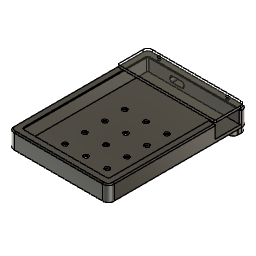
FudaBako (Autodesk Fusion 360 design; units mm, degrees)
Autodesk Fusion 360 part; units mm, degrees
sketch "スケッチ1" plane through (0, 0, 0) normal (0, 0, 1) x (1, 0, 0)
  line L0 (0, 0) -> (72, 0)
  line L1 (72, 0) -> (72, 105.5)
  line L2 (72, 105.5) -> (0, 105.5)
  line L3 (0, 105.5) -> (0, 0)
  line L4 (0, 0) -> (72, 0)
  line L5 (72, 0) -> (72, 85)
  line L6 (72, 85) -> (0, 85)
  line L7 (0, 85) -> (0, 0)
  line L8 (-0.5, -0.5) -> (72.5, -0.5)
  line L9 (72.5, -0.5) -> (72.5, 106)
  line L10 (72.5, 106) -> (-0.5, 106)
  line L11 (-0.5, 106) -> (-0.5, -0.5)
  line L12 (-6.5, -6.5) -> (78.5, -6.5)
  line L13 (78.5, -6.5) -> (78.5, 112)
  line L14 (78.5, 112) -> (-6.5, 112)
  line L15 (-6.5, 112) -> (-6.5, -6.5)
  dimension "d1" = 72
  dimension "d2" = 105.5
  dimension "d3" = 72
  dimension "d4" = 85
  dimension "d5" = 0.5
  dimension "d6" = 0.5
  dimension "d7" = 0.5
  dimension "d8" = 0.5
  dimension "d9" = 6
  dimension "d10" = 6
  dimension "d11" = 6
  dimension "d12" = 6
  constraint horizontal L0
  constraint vertical L1
  constraint horizontal L2
  constraint vertical L3
  constraint coincident L0.start L3.end
  constraint horizontal L4
  constraint vertical L5
  constraint horizontal L6
  constraint vertical L7
  constraint horizontal L8
  constraint vertical L9
  constraint horizontal L10
  constraint vertical L11
  constraint horizontal L12
  constraint vertical L13
  constraint horizontal L14
  constraint vertical L15
  measures "d1" distance of L0.start L0.end
  measures "d2" distance of L0.start L2.end
  measures "d3" distance of L0.start L0.end
  measures "d4" distance of L0.start L6.end
  measures "d5" distance of L2 L10
  measures "d6" distance of L3 L11
  measures "d7" distance of L1 L9
  measures "d8" distance of L4 L8
  measures "d9" distance of L10 L14
  measures "d10" distance of L8 L12
  measures "d11" distance of L9 L13
  measures "d12" distance of L11 L15
extrude "押し出し1" add sketch "スケッチ1" along normal blind 14 contours L12 L13 L14 L15 makes body 1
extrude "押し出し2" add sketch "スケッチ1" 1 faces at (-4.5, 70.5, 0) along normal blind 3 contours L0 L1 L3 L4 L5 L6 L7 | L1 L2 L3 L6 | L8 L9 L10 L11 | L12 L13 L14 L15 on bodies 1 bodies 1
sketch "スケッチ2" plane through (0, 0, 14) normal (0, 0, 1) x (-1, 0, 0)
  line L0 (-72.5, 0.5) -> (0.5, 0.5)
  line L1 (6.5, 6.5) -> (-78.5, 6.5)
  line L2 (-78.5, -112) -> (6.5, -112)
  line L3 (-78.5, -112) -> (6.5, -112)
  line L4 (6.5, -112) -> (6.5, 6.5)
  line L5 (6.5, -85.5) -> (-78.5, -85.5)
  line L6 (-78.5, -85.5) -> (-78.5, -112)
  line L7 (-78.5, -112) -> (6.5, -112)
  line L8 (6.5, -112) -> (6.5, -85.5)
  line L9 (0.5, -106) -> (-72.5, -106)
  line L10 (-72.5, -106) -> (-72.5, -85.5)
  line L11 (-72.5, -85.5) -> (0.5, -85.5)
  line L12 (0.5, -85.5) -> (0.5, -106)
  line L13 (0.5, -106) -> (6.5, -106)
  line L14 (6.5, -106) -> (6.5, -85.5)
  line L15 (6.5, -85.5) -> (0.5, -85.5)
  line L16 (0.5, -85.5) -> (0.5, -106)
  line L17 (-72.5, -106) -> (-78.5, -106)
  line L18 (-78.5, -106) -> (-78.5, -85.5)
  line L19 (-78.5, -85.5) -> (-72.5, -85.5)
  line L20 (-72.5, -85.5) -> (-72.5, -106)
  point P0 (-72.5, -106)
  point P1 (0.5, -106)
  dimension "d190" = 20.5
  constraint coincident L5.start L4
  constraint horizontal L5
  constraint vertical L6
  constraint horizontal L7
  constraint vertical L8
  constraint coincident L2.start L3.start
  constraint horizontal L9
  constraint vertical L10
  constraint horizontal L11
  constraint vertical L12
  constraint coincident L5 L10.end
  constraint coincident P0 L9.end
  constraint coincident P1 L9.start
  constraint horizontal L13
  constraint vertical L14
  constraint horizontal L15
  constraint vertical L16
  constraint horizontal L17
  constraint vertical L18
  constraint horizontal L19
  constraint vertical L20
  measures "d190" distance of P1 L11.end
extrude "押し出し4" cut sketch "スケッチ2" against normal blind 11 contours L5 L6 L10 L17 L18 L19 L20 bodies 1
sketch "スケッチ6" plane through (0, 0, 3) normal (0, 0, 1) x (-1, 0, 0)
  line L0 (0.5, 0.5) -> (-72.5, 0.5)
  line L1 (-72.5, 0.5) -> (-72.5, -85.5)
  line L2 (0.5, -106) -> (0.5, 0.5)
  circle A0 centre (-18, -68) radius 1.1
  line L3 (-72, -85) -> (0, -85)
  line L4 (0, -105.5) -> (0, 0)
  circle A1 centre (-54, -68) radius 1.1
  line L5 (-72, 0) -> (-72, -85)
  circle A2 centre (-36, -51) radius 1.1
  circle A3 centre (-18, -51) radius 1.1
  circle A4 centre (-54, -51) radius 1.1
  circle A5 centre (-36, -68) radius 1.1
  circle A6 centre (-18, -34) radius 1.1
  circle A7 centre (-36, -34) radius 1.1
  circle A8 centre (-54, -34) radius 1.1
  circle A9 centre (-36, -17) radius 1.1
  circle A10 centre (-18, -17) radius 1.1
  circle A11 centre (-54, -17) radius 1.1
  line L6 (0, -85) -> (0, 0)
  line L7 (0, 0) -> (-72, 0)
  circle A12 centre (-56.5, -4) radius 1.1
  line L8 (-72.5, -85.5) -> (-78.5, -85.5)
  line L9 (-78.5, -85.5) -> (-78.5, -106)
  line L10 (-78.5, -106) -> (0.5, -106)
  circle A13 centre (-15.5, -4) radius 1.1
  dimension "d45" = 2.2
  dimension "d46" = 17
  dimension "d47" = 18
  dimension "d48" = 2.2
  dimension "d49" = 17
  dimension "d50" = 18
  dimension "d51" = 2.2
  dimension "d52" = 34
  dimension "d53" = 36
  dimension "d54" = 2.2
  dimension "d55" = 18
  dimension "d56" = 34
  dimension "d57" = 2.2
  dimension "d58" = 2.2
  dimension "d59" = 17
  dimension "d60" = 36
  dimension "d61" = 18
  dimension "d62" = 34
  dimension "d63" = 2.2
  dimension "d64" = 2.2
  dimension "d65" = 2.2
  dimension "d66" = 2.2
  dimension "d67" = 2.2
  dimension "d68" = 2.2
  dimension "d69" = 18
  dimension "d70" = 36
  dimension "d71" = 18
  dimension "d72" = 34
  dimension "d73" = 17
  dimension "d74" = 18
  dimension "d75" = 36
  dimension "d76" = 17
  dimension "d77" = 34
  dimension "d78" = 34
  dimension "d79" = 18
  dimension "d80" = 17
  dimension "d81" = 2.2
  dimension "d82" = 15.5
  dimension "d83" = 4
  dimension "d268" = 2.2
  dimension "d269" = 15.5
  dimension "d270" = 4
  measures "d45" diameter of A0
  measures "d46" distance of A0.centre L3
  measures "d47" distance of A0.centre L4
  measures "d48" diameter of A1
  measures "d49" distance of L3 A1.centre
  measures "d50" distance of A1.centre L5
  measures "d51" diameter of A2
  measures "d52" distance of L3 A2.centre
  measures "d53" distance of L4 A2.centre
  measures "d54" diameter of A3
  measures "d55" distance of L4 A3.centre
  measures "d56" distance of L3 A3.centre
  measures "d57" diameter of A4
  measures "d58" diameter of A5
  measures "d59" distance of L3 A5.centre
  measures "d60" distance of L4 A5.centre
  measures "d61" distance of L5 A4.centre
  measures "d62" distance of L3 A4.centre
  measures "d63" diameter of A7
  measures "d64" diameter of A6
  measures "d65" diameter of A8
  measures "d66" diameter of A9
  measures "d67" diameter of A10
  measures "d68" diameter of A11
  measures "d69" distance of L5 A8.centre
  measures "d70" distance of A7.centre L6
  measures "d71" distance of A6.centre L6
  measures "d72" distance of A6.centre L7
  measures "d73" distance of A10.centre L7
  measures "d74" distance of A10.centre L6
  measures "d75" distance of A9.centre L6
  measures "d76" distance of A9.centre L7
  measures "d77" distance of A7.centre L7
  measures "d78" distance of A8.centre L7
  measures "d79" distance of L5 A11.centre
  measures "d80" distance of A11.centre L7
  measures "d81" diameter of A12
  measures "d82" distance of L5 A12.centre
  measures "d83" distance of L7 A12.centre
  measures "d268" diameter of A13
  measures "d269" distance of L6 A13.centre
  measures "d270" distance of L7 A13.centre
extrude "押し出し8" cut sketch "スケッチ6" against normal blind 3 contours A0 | A1 | A2 | A3 | A4 | A5 | A6 | A7 | A8 | A9 | A10 | A11 | A12 | A13 bodies 1
sketch "スケッチ7" plane through (0, 0, 3) normal (0, 0, 1) x (-1, 0, 0)
  circle A0 centre (-54, -17) radius 1.1
  circle A1 centre (-18, -34) radius 1.1
  circle A2 centre (-54, -68) radius 1.1
  circle A3 centre (-36, -68) radius 1.1
  circle A4 centre (-18, -51) radius 1.1
  circle A5 centre (-36, -17) radius 1.1
  circle A6 centre (-54, -34) radius 1.1
  circle A7 centre (-36, -34) radius 1.1
  circle A8 centre (-54, -51) radius 1.1
  circle A9 centre (-18, -68) radius 1.1
  circle A10 centre (-36, -51) radius 1.1
  circle A11 centre (-18, -17) radius 1.1
  circle A12 centre (-56.5, -4) radius 1.1
  line L0 (0.5, 0.5) -> (-72.5, 0.5)
  line L1 (-72.5, 0.5) -> (-72.5, -85.5)
  line L2 (0.5, -106) -> (0.5, 0.5)
  circle A13 centre (-18, -68) radius 2.1
  circle A14 centre (-36, -68) radius 2.1
  circle A15 centre (-54, -68) radius 2.1
  circle A16 centre (-18, -51) radius 2.1
  circle A17 centre (-36, -51) radius 2.1
  circle A18 centre (-54, -51) radius 2.1
  circle A19 centre (-54, -34) radius 2.1
  circle A20 centre (-54, -17) radius 2.1
  circle A21 centre (-56.5, -4) radius 2.1
  circle A22 centre (-36, -34) radius 2.1
  circle A23 centre (-18, -34) radius 2.1
  circle A24 centre (-18, -17) radius 2.1
  circle A25 centre (-36, -17) radius 2.1
  line L3 (-72.5, -85.5) -> (-78.5, -85.5)
  line L4 (-78.5, -85.5) -> (-78.5, -106)
  line L5 (-78.5, -106) -> (0.5, -106)
  circle A26 centre (-15.5, -4) radius 1.1
  circle A27 centre (-15.5, -4) radius 2.1
  dimension "d86" = 4.2
  dimension "d87" = 4.2
  dimension "d88" = 4.2
  dimension "d89" = 4.2
  dimension "d90" = 4.2
  dimension "d91" = 4.2
  dimension "d92" = 4.2
  dimension "d93" = 4.2
  dimension "d94" = 4.2
  dimension "d95" = 4.2
  dimension "d96" = 4.2
  dimension "d97" = 4.2
  dimension "d98" = 4.2
  dimension "d272" = 4.2
  constraint concentric A9 A13
  constraint concentric A3 A14
  constraint concentric A2 A15
  constraint concentric A4 A16
  constraint concentric A10 A17
  constraint concentric A8 A18
  constraint concentric A6 A19
  constraint concentric A0 A20
  constraint concentric A12 A21
  constraint concentric A7 A22
  constraint concentric A1 A23
  constraint concentric A11 A24
  constraint concentric A5 A25
  constraint concentric A26 A27
  measures "d86" diameter of A13
  measures "d87" diameter of A14
  measures "d88" diameter of A15
  measures "d89" diameter of A16
  measures "d90" diameter of A17
  measures "d91" diameter of A18
  measures "d92" diameter of A19
  measures "d93" diameter of A20
  measures "d94" diameter of A21
  measures "d95" diameter of A22
  measures "d96" diameter of A23
  measures "d97" diameter of A24
  measures "d98" diameter of A25
  measures "d272" diameter of A27
extrude "押し出し9" cut sketch "スケッチ7" against normal blind 1 contours A13 | A14 | A15 | A16 | A17 | A18 | A19 | A20 | A21 | A22 | A23 | A24 | A25 | A27 bodies 1
sketch "スケッチ8" plane through (0, 0, 0) normal (0, 0, 1) x (1, 0, 0)
  circle A0 centre (72.5, -0.5) radius 3.75
  line L0 (78.5, -6.5) -> (78.5, 112)
  line L1 (-6.5, -6.5) -> (78.5, -6.5)
  circle A1 centre (-0.5, -0.5) radius 3.75
  line L2 (-6.5, 112) -> (-6.5, -6.5)
  circle A2 centre (72.5, 106) radius 3.75
  line L3 (78.5, 112) -> (-6.5, 112)
  circle A3 centre (-0.5, 106) radius 3.75
  dimension "d101" = 7.5
  dimension "d102" = 6
  dimension "d103" = 6
  dimension "d104" = 7.5
  dimension "d105" = 6
  dimension "d106" = 6
  dimension "d107" = 7.5
  dimension "d108" = 6
  dimension "d109" = 6
  dimension "d110" = 7.5
  dimension "d111" = 6
  dimension "d112" = 6
  measures "d101" diameter of A0
  measures "d102" distance of A0.centre L0
  measures "d103" distance of A0.centre L1
  measures "d104" diameter of A1
  measures "d105" distance of L1 A1.centre
  measures "d106" distance of A1.centre L2
  measures "d107" diameter of A2
  measures "d108" distance of L0 A2.centre
  measures "d109" distance of A2.centre L3
  measures "d110" diameter of A3
  measures "d111" distance of L2 A3.centre
  measures "d112" distance of L3 A3.centre
extrude "押し出し10" cut sketch "スケッチ8" along normal blind 0.5 contours A0 | A1 | A2 | A3 bodies 1
sketch "スケッチ10" plane through (0, 0, 0) normal (0, 0, -1) x (1, 0, 0)
  circle A0 centre (56.5, -4) radius 1.1
  circle A1 centre (18, -17) radius 1.1
  circle A2 centre (36, -51) radius 1.1
  circle A3 centre (18, -68) radius 1.1
  circle A4 centre (54, -51) radius 1.1
  circle A5 centre (36, -34) radius 1.1
  circle A6 centre (54, -34) radius 1.1
  circle A7 centre (36, -17) radius 1.1
  circle A8 centre (18, -51) radius 1.1
  circle A9 centre (36, -68) radius 1.1
  circle A10 centre (54, -68) radius 1.1
  circle A11 centre (18, -34) radius 1.1
  circle A12 centre (54, -17) radius 1.1
  circle A13 centre (72.5, 0.5) radius 3.75
  circle A14 centre (-0.5, 0.5) radius 3.75
  circle A15 centre (56.5, -4) radius 2
  circle A16 centre (54, -17) radius 2
  circle A17 centre (36, -17) radius 2
  circle A18 centre (18, -17) radius 2
  circle A19 centre (18, -34) radius 2
  circle A20 centre (36, -34) radius 2
  circle A21 centre (54, -34) radius 2
  circle A22 centre (54, -51) radius 2
  circle A23 centre (36, -51) radius 2
  circle A24 centre (18, -51) radius 2
  circle A25 centre (18, -68) radius 2
  circle A26 centre (36, -68) radius 2
  circle A27 centre (54, -68) radius 2
  line L0 (-6.5, 6.5) -> (-6.5, -112)
  line L1 (78.5, -112) -> (78.5, 6.5)
  line L2 (78.5, 6.5) -> (-6.5, 6.5)
  circle A28 centre (-0.5, -106) radius 3.75
  circle A29 centre (72.5, -106) radius 3.75
  line L3 (-6.5, -112) -> (78.5, -112)
  circle A30 centre (15.5, -4) radius 1.1
  circle A31 centre (15.5, -4) radius 2
  dimension "d135" = 4
  dimension "d136" = 4
  dimension "d137" = 4
  dimension "d138" = 4
  dimension "d139" = 4
  dimension "d140" = 4
  dimension "d141" = 4
  dimension "d142" = 4
  dimension "d143" = 4
  dimension "d144" = 4
  dimension "d145" = 4
  dimension "d146" = 4
  dimension "d147" = 4
  dimension "d271" = 4
  constraint concentric A0 A15
  constraint concentric A12 A16
  constraint concentric A7 A17
  constraint concentric A1 A18
  constraint concentric A11 A19
  constraint concentric A5 A20
  constraint concentric A6 A21
  constraint concentric A4 A22
  constraint concentric A2 A23
  constraint concentric A8 A24
  constraint concentric A3 A25
  constraint concentric A9 A26
  constraint concentric A10 A27
  constraint concentric A30 A31
  measures "d135" diameter of A15
  measures "d136" diameter of A16
  measures "d137" diameter of A17
  measures "d138" diameter of A18
  measures "d139" diameter of A19
  measures "d140" diameter of A20
  measures "d141" diameter of A21
  measures "d142" diameter of A22
  measures "d143" diameter of A23
  measures "d144" diameter of A24
  measures "d145" diameter of A25
  measures "d146" diameter of A26
  measures "d147" diameter of A27
  measures "d271" diameter of A31
extrude "押し出し13" cut sketch "スケッチ10" against normal blind 0.5 contours A15 | A16 | A17 | A18 | A19 | A20 | A21 | A22 | A23 | A24 | A25 | A26 | A27 | A31 bodies 1
fillet "フィレット4" radius 1 2 edges at (72.5, -0.5, 8.5) (-0.5, -0.5, 8.5) on bodies 1
fillet "フィレット16" radius 1 1 edges at (-0.5, 106, 8.5) on bodies 1
chamfer "面取り12" distance 0.5 angle 45 5 edges at (72.5, 43, 14) (72.2071, -0.2071, 14) (36, -0.5, 14) (-0.2071, -0.2071, 14) (-0.5, 53.25, 14) on bodies 1
fillet "フィレット5" radius 5 curvature continuous 2 edges at (78.5, -6.5, 7) (-6.5, -6.5, 7) on bodies 1
fillet "フィレット8" radius 1 1 edges at (78.5, 85.5, 8.5) on bodies 1
fillet "フィレット13" radius 5 curvature continuous 2 edges at (78.5, 112, 7) (-6.5, 112, 7) on bodies 1
chamfer "面取り21" distance 1 angle 45 12 edges at (36, 112, 14) (77.0839, 110.8219, 14) (78.5, 106.75, 14) (78.5, 41.5, 14) (75.25, 85.5, 14) (78.2071, 85.2071, 14) (78.5, 41.5, 14) (77.3219, -5.0839, 14) (36, -6.5, 14) (-5.0839, -5.3219, 14) (-6.5, 52.75, 14) (-5.3219, 110.5839, 14) on bodies 1
fillet "フィレット15" radius 1 2 edges at (72.5, 85.5, 8) (78.5, 106, 8) on bodies 1
sketch "スケッチ17" plane through (0, 0, 14) normal (0, 0, 1) x (-1, 0, 0)
  line L0 (-77.5, -106.5) -> (-77.5, -107)
  line L1 (-73.5, -111) -> (1.5, -111)
  line L2 (5.5, -107) -> (5.5, 1.5)
  circle A0 centre (-7, -108.5) radius 0.9
  circle A1 centre (-65, -108.5) radius 0.9
  line L3 (-73.5, -112) -> (1.5, -112)
  spline S0 degree 3 poles (-73.5, -111) (-73.8454, -111) (-74.1654, -110.9986) (-74.7027, -110.9408) (-74.9267, -110.8989) (-75.2988, -110.7824) (-75.4373, -110.7274) (-75.8631, -110.522) (-76.1365, -110.3374) (-76.4029, -110.0896) (-76.6724, -109.839) (-76.9308, -109.521) (-77.3045, -108.8015) (-77.3918, -108.4745) (-77.4569, -108.0594) (-77.4694, -107.9483) (-77.4991, -107.5718) (-77.5, -107.2964) (-77.5, -107) knots 0 0 0 0 0.103632 0.103632 0.182254 0.182254 0.2323 0.2323 0.339984 0.339984 0.339984 0.448922 0.448922 0.55397 0.55397 0.591904 0.591904 0.679968 0.679968 0.679968 0.679968
  spline S1 degree 3 poles (5.5, -107) (5.5, -107.3454) (5.4986, -107.6654) (5.4408, -108.2027) (5.3989, -108.4267) (5.2824, -108.7988) (5.2274, -108.9373) (5.022, -109.3631) (4.8374, -109.6365) (4.5896, -109.9029) (4.339, -110.1724) (4.021, -110.4308) (3.3015, -110.8045) (2.9745, -110.8918) (2.5594, -110.9569) (2.4483, -110.9694) (2.0718, -110.9991) (1.7964, -111) (1.5, -111) knots 0 0 0 0 0.103632 0.103632 0.182254 0.182254 0.2323 0.2323 0.339984 0.339984 0.339984 0.448922 0.448922 0.55397 0.55397 0.591904 0.591904 0.679968 0.679968 0.679968 0.679968
  line L4 (1, -0.5) -> (1, -105)
  spline S2 degree 3 poles (1.5, 5.5) (1.8454, 5.5) (2.1654, 5.4986) (2.7027, 5.4408) (2.9267, 5.3989) (3.2988, 5.2824) (3.4373, 5.2274) (3.8631, 5.022) (4.1365, 4.8374) (4.4029, 4.5896) (4.6724, 4.339) (4.9308, 4.021) (5.3045, 3.3015) (5.3918, 2.9745) (5.4569, 2.5594) (5.4694, 2.4483) (5.4991, 2.0718) (5.5, 1.7964) (5.5, 1.5) knots 0 0 0 0 0.103632 0.103632 0.182254 0.182254 0.2323 0.2323 0.339984 0.339984 0.339984 0.448922 0.448922 0.55397 0.55397 0.591904 0.591904 0.679968 0.679968 0.679968 0.679968
  line L5 (1.5, 5.5) -> (-73.5, 5.5)
  spline S3 degree 3 poles (-77.5, 1.5) (-77.5, 1.8454) (-77.4986, 2.1654) (-77.4408, 2.7027) (-77.3989, 2.9267) (-77.2824, 3.2988) (-77.2274, 3.4373) (-77.022, 3.8631) (-76.8374, 4.1365) (-76.5896, 4.4029) (-76.339, 4.6724) (-76.021, 4.9308) (-75.3015, 5.3045) (-74.9745, 5.3918) (-74.5594, 5.4569) (-74.4483, 5.4694) (-74.0718, 5.4991) (-73.7964, 5.5) (-73.5, 5.5) knots 0 0 0 0 0.103632 0.103632 0.182254 0.182254 0.2323 0.2323 0.339984 0.339984 0.339984 0.448922 0.448922 0.55397 0.55397 0.591904 0.591904 0.679968 0.679968 0.679968 0.679968
  line L6 (-77.5, 1.5) -> (-77.5, -84.5)
  line L7 (-77.5, -84.5) -> (-73, -84.5)
  line L8 (-73, -84.5) -> (-73, -0.5)
  arc A2 (-71.5, 1) -> (-73, -0.5) centre (-71.5, -0.5) ccw
  line L9 (-71.5, 1) -> (-0.5, 1)
  arc A3 (1, -0.5) -> (-0.5, 1) centre (-0.5, -0.5) ccw
  arc A4 (-0.5, -106.5) -> (1, -105) centre (-0.5, -105) ccw
  line L10 (-0.5, -106.5) -> (-77.5, -106.5)
  point P0 (-78.5, -107)
  point P1 (6.5, -107)
  dimension "d236" = 1.8
  dimension "d237" = 1.8
  dimension "d238" = 13.5
  dimension "d240" = 3.5
  dimension "d241" = 3.5
  measures "d236" diameter of A0
  measures "d237" diameter of A1
  measures "d238" horizontal distance of A1.centre P0
  measures "d240" distance of A0.centre L3
  measures "d241" distance of A1.centre L3
extrude "押し出し22" cut sketch "スケッチ17" against normal blind 6 contours A0 | A1 bodies 1
sketch "スケッチ18" plane through (0, 112, 0) normal (0, 1, 0) x (-1, 0, 0)
  line L0 (1.5, 13) -> (-73.5, 13)
  line L1 (-73.5, 13) -> (-73.5, 0)
  line L2 (-73.5, 0) -> (1.5, 0)
  line L3 (1.5, 0) -> (1.5, 13)
  line L4 (-51.5, 10.1) -> (-43.5, 10.1)
  line L5 (-41.5, 8.1) -> (-41.5, 7.1)
  line L6 (-43.5, 5.1) -> (-51.5, 5.1)
  line L7 (-53.5, 7.1) -> (-53.5, 8.1)
  line L8 (-28.5, 10.1) -> (-20.5, 10.1)
  line L9 (-18.5, 8.1) -> (-18.5, 7.1)
  line L10 (-20.5, 5.1) -> (-28.5, 5.1)
  line L11 (-30.5, 7.1) -> (-30.5, 8.1)
  line L12 (-78.5, 13) -> (-78.5, 3)
  arc A0 (-51.5, 10.1) -> (-53.5, 8.1) centre (-51.5, 8.1) ccw
  arc A1 (-53.5, 7.1) -> (-51.5, 5.1) centre (-51.5, 7.1) ccw
  arc A2 (-41.5, 8.1) -> (-43.5, 10.1) centre (-43.5, 8.1) ccw
  arc A3 (-43.5, 5.1) -> (-41.5, 7.1) centre (-43.5, 7.1) ccw
  arc A4 (-28.5, 10.1) -> (-30.5, 8.1) centre (-28.5, 8.1) ccw
  arc A5 (-30.5, 7.1) -> (-28.5, 5.1) centre (-28.5, 7.1) ccw
  arc A6 (-18.5, 8.1) -> (-20.5, 10.1) centre (-20.5, 8.1) ccw
  arc A7 (-20.5, 5.1) -> (-18.5, 7.1) centre (-20.5, 7.1) ccw
  line L13 (6.5, 0) -> (6.5, 13)
  point P0 (-53.5, 10.1)
  point P1 (-41.5, 10.1)
  point P2 (-53.5, 5.1)
  point P3 (-30.5, 10.1)
  point P4 (-18.5, 10.1)
  point P5 (-18.5, 5.1)
  point P6 (-30.5, 5.1)
  dimension "d244" = 25
  dimension "d246" = 12
  dimension "d247" = 12
  dimension "d248" = 5
  dimension "d249" = 5
  dimension "d250" = 5.1
  dimension "d251" = 5.1
  dimension "d252" = 2
  dimension "d253" = 2
  dimension "d254" = 2
  dimension "d255" = 2
  dimension "d256" = 2
  dimension "d257" = 2
  dimension "d258" = 2
  dimension "d259" = 2
  dimension "d282" = 25
  constraint horizontal L4
  constraint vertical L5
  constraint horizontal L6
  constraint vertical L7
  constraint horizontal L8
  constraint vertical L9
  constraint horizontal L10
  constraint vertical L11
  constraint coincident P0 L4
  constraint coincident P0 L7
  constraint tangent L4 A0
  constraint tangent L7 A0
  constraint coincident P2 L6
  constraint coincident P2 L7
  constraint tangent L6 A1
  constraint tangent L7 A1
  constraint coincident P1 L4
  constraint coincident P1 L5
  constraint tangent L4 A2
  constraint tangent L5 A2
  constraint tangent L5 A3
  constraint tangent L6 A3
  constraint coincident P3 L8
  constraint coincident P3 L11
  constraint tangent L8 A4
  constraint tangent L11 A4
  constraint coincident P6 L10
  constraint coincident P6 L11
  constraint tangent L10 A5
  constraint tangent L11 A5
  constraint coincident P4 L8
  constraint coincident P4 L9
  constraint tangent L8 A6
  constraint tangent L9 A6
  constraint coincident P5 L9
  constraint coincident P5 L10
  constraint tangent L9 A7
  constraint tangent L10 A7
  measures "d244" distance of L7 L12
  measures "d246" distance of P3 P4
  measures "d247" distance of P0 P1
  measures "d248" distance of P0 P2
  measures "d249" distance of P4 P5
  measures "d250" distance of L2 P6
  measures "d251" distance of L2 P2
  measures "d252" radius of A0
  measures "d253" radius of A1
  measures "d254" radius of A2
  measures "d255" radius of A3
  measures "d256" radius of A4
  measures "d257" radius of A5
  measures "d258" radius of A6
  measures "d259" radius of A7
  measures "d282" distance of L9.start L13
extrude "押し出し23" cut sketch "スケッチ18" against normal blind 7 contours L8 L9 L10 L11 A4 A5 A6 A7 bodies 1
chamfer "面取り22" distance 1 angle 45 8 edges at (24.5, 112, 10.1) (19.0858, 112, 9.5142) (18.5, 112, 7.6) (19.0858, 112, 5.6858) (24.5, 112, 5.1) (29.9142, 112, 5.6858) (30.5, 112, 7.6) (29.9142, 112, 9.5142) on bodies 1
sketch "スケッチ19" plane through (0, 0, 14) normal (0, 0, 1) x (-1, 0, 0)
  circle A0 centre (-7, -108.5) radius 0.9
  circle A1 centre (-65, -108.5) radius 0.9
  line L0 (-77.5, -106.5) -> (-77.5, -107)
  line L1 (-73.5, -111) -> (1.5, -111)
  line L2 (5.5, -107) -> (5.5, 1.5)
  line L3 (5.5, -107) -> (-77.5, -107)
  line L4 (-77.5, -107) -> (-77.5, -86.5)
  line L5 (-76.5, -85.5) -> (4.5, -85.5)
  line L6 (5.5, -86.5) -> (5.5, -107)
  arc A2 (-76.5, -85.5) -> (-77.5, -86.5) centre (-76.5, -86.5) ccw
  arc A3 (5.5, -86.5) -> (4.5, -85.5) centre (4.5, -86.5) ccw
  spline S0 degree 3 poles (-73.5, -111) (-73.8454, -111) (-74.1654, -110.9986) (-74.7027, -110.9408) (-74.9267, -110.8989) (-75.2988, -110.7824) (-75.4373, -110.7274) (-75.8631, -110.522) (-76.1365, -110.3374) (-76.4029, -110.0896) (-76.6724, -109.839) (-76.9308, -109.521) (-77.3045, -108.8015) (-77.3918, -108.4745) (-77.4569, -108.0594) (-77.4694, -107.9483) (-77.4991, -107.5718) (-77.5, -107.2964) (-77.5, -107) knots 0 0 0 0 0.103632 0.103632 0.182254 0.182254 0.2323 0.2323 0.339984 0.339984 0.339984 0.448922 0.448922 0.55397 0.55397 0.591904 0.591904 0.679968 0.679968 0.679968 0.679968
  spline S1 degree 3 poles (5.5, -107) (5.5, -107.3454) (5.4986, -107.6654) (5.4408, -108.2027) (5.3989, -108.4267) (5.2824, -108.7988) (5.2274, -108.9373) (5.022, -109.3631) (4.8374, -109.6365) (4.5896, -109.9029) (4.339, -110.1724) (4.021, -110.4308) (3.3015, -110.8045) (2.9745, -110.8918) (2.5594, -110.9569) (2.4483, -110.9694) (2.0718, -110.9991) (1.7964, -111) (1.5, -111) knots 0 0 0 0 0.103632 0.103632 0.182254 0.182254 0.2323 0.2323 0.339984 0.339984 0.339984 0.448922 0.448922 0.55397 0.55397 0.591904 0.591904 0.679968 0.679968 0.679968 0.679968
  line L7 (1, -0.5) -> (1, -105)
  spline S2 degree 3 poles (1.5, 5.5) (1.8454, 5.5) (2.1654, 5.4986) (2.7027, 5.4408) (2.9267, 5.3989) (3.2988, 5.2824) (3.4373, 5.2274) (3.8631, 5.022) (4.1365, 4.8374) (4.4029, 4.5896) (4.6724, 4.339) (4.9308, 4.021) (5.3045, 3.3015) (5.3918, 2.9745) (5.4569, 2.5594) (5.4694, 2.4483) (5.4991, 2.0718) (5.5, 1.7964) (5.5, 1.5) knots 0 0 0 0 0.103632 0.103632 0.182254 0.182254 0.2323 0.2323 0.339984 0.339984 0.339984 0.448922 0.448922 0.55397 0.55397 0.591904 0.591904 0.679968 0.679968 0.679968 0.679968
  line L8 (1.5, 5.5) -> (-73.5, 5.5)
  spline S3 degree 3 poles (-77.5, 1.5) (-77.5, 1.8454) (-77.4986, 2.1654) (-77.4408, 2.7027) (-77.3989, 2.9267) (-77.2824, 3.2988) (-77.2274, 3.4373) (-77.022, 3.8631) (-76.8374, 4.1365) (-76.5896, 4.4029) (-76.339, 4.6724) (-76.021, 4.9308) (-75.3015, 5.3045) (-74.9745, 5.3918) (-74.5594, 5.4569) (-74.4483, 5.4694) (-74.0718, 5.4991) (-73.7964, 5.5) (-73.5, 5.5) knots 0 0 0 0 0.103632 0.103632 0.182254 0.182254 0.2323 0.2323 0.339984 0.339984 0.339984 0.448922 0.448922 0.55397 0.55397 0.591904 0.591904 0.679968 0.679968 0.679968 0.679968
  line L9 (-77.5, 1.5) -> (-77.5, -84.5)
  line L10 (-77.5, -84.5) -> (-73, -84.5)
  line L11 (-73, -84.5) -> (-73, -0.5)
  arc A4 (-71.5, 1) -> (-73, -0.5) centre (-71.5, -0.5) ccw
  line L12 (-71.5, 1) -> (-0.5, 1)
  arc A5 (1, -0.5) -> (-0.5, 1) centre (-0.5, -0.5) ccw
  arc A6 (-0.5, -106.5) -> (1, -105) centre (-0.5, -105) ccw
  line L13 (-0.5, -106.5) -> (-77.5, -106.5)
  dimension "d264" = 1
  dimension "d265" = 1
  constraint horizontal L3
  constraint vertical L4
  constraint horizontal L5
  constraint vertical L6
  constraint coincident L0.start L4
  constraint coincident L2.start L3
  constraint tangent L4 A2
  constraint tangent L5 A2
  constraint tangent L5 A3
  constraint tangent L6 A3
  measures "d264" radius of A2
  measures "d265" radius of A3
extrude "押し出し24" add sketch "スケッチ19" along normal blind 2 separate body contours L0 L2 L3 L4 L5 L6 A3 L7 A6 L13 | L4 L5 A2 L7 A6 L13 | L1 L3 S0 S1 makes body 2
sketch "スケッチ20" plane through (0, 0, 0) normal (0, 0, -1) x (1, 0, 0)
  line L0 (-1.5, -112) -> (73.5, -112)
  line L1 (78.5, -107) -> (78.5, 1.5)
  line L2 (73.5, 6.5) -> (-1.5, 6.5)
  line L3 (-6.5, 1.5) -> (-6.5, -107)
  circle A0 centre (72.5, 0.5) radius 3.75
  circle A1 centre (72.5, -106) radius 3.75
  circle A2 centre (-0.5, 0.5) radius 3.75
  circle A3 centre (-0.5, -106) radius 3.75
  circle A4 centre (15.5, -4) radius 2
  circle A5 centre (18, -51) radius 2
  circle A6 centre (36, -34) radius 2
  circle A7 centre (54, -17) radius 2
  circle A8 centre (36, -17) radius 2
  circle A9 centre (54, -34) radius 2
  circle A10 centre (18, -68) radius 2
  circle A11 centre (54, -68) radius 2
  circle A12 centre (36, -51) radius 2
  circle A13 centre (18, -34) radius 2
  circle A14 centre (56.5, -4) radius 2
  circle A15 centre (18, -17) radius 2
  circle A16 centre (54, -51) radius 2
  circle A17 centre (36, -68) radius 2
  circle A18 centre (58.5, -108.5) radius 0.9
  circle A19 centre (13.5, -108.5) radius 0.9
  spline S0 degree 3 poles (73.5, 6.5) (74.1075, 6.5) (74.7567, 6.5) (75.9834, 6.1158) (76.4633, 5.8499) (77.3109, 5.1398) (77.7145, 4.6816) (78.2502, 3.6503) (78.3672, 3.2095) (78.5, 2.3629) (78.5, 1.9241) (78.5, 1.5) knots 0 0 0 0 0.182254 0.182254 0.32114 0.32114 0.448922 0.448922 0.55397 0.55397 0.679968 0.679968 0.679968 0.679968
  spline S1 degree 3 poles (-6.5, 1.5) (-6.5, 2.1075) (-6.5, 2.7567) (-6.1158, 3.9834) (-5.8499, 4.4633) (-5.1398, 5.3109) (-4.6816, 5.7145) (-3.6503, 6.2502) (-3.2095, 6.3672) (-2.3629, 6.5) (-1.9241, 6.5) (-1.5, 6.5) knots 0 0 0 0 0.182254 0.182254 0.32114 0.32114 0.448922 0.448922 0.55397 0.55397 0.679968 0.679968 0.679968 0.679968
  spline S2 degree 3 poles (-1.5, -112) (-2.1075, -112) (-2.7567, -112) (-3.9834, -111.6158) (-4.4633, -111.3499) (-5.3109, -110.6398) (-5.7145, -110.1816) (-6.2502, -109.1503) (-6.3672, -108.7095) (-6.5, -107.8629) (-6.5, -107.4241) (-6.5, -107) knots 0 0 0 0 0.182254 0.182254 0.32114 0.32114 0.448922 0.448922 0.55397 0.55397 0.679968 0.679968 0.679968 0.679968
  spline S3 degree 3 poles (78.5, -107) (78.5, -107.6075) (78.5, -108.2567) (78.1158, -109.4834) (77.8499, -109.9633) (77.1398, -110.8109) (76.6816, -111.2145) (75.6503, -111.7502) (75.2095, -111.8672) (74.3629, -112) (73.9241, -112) (73.5, -112) knots 0 0 0 0 0.182254 0.182254 0.32114 0.32114 0.448922 0.448922 0.55397 0.55397 0.679968 0.679968 0.679968 0.679968
  dimension "d273" = 1.8
  dimension "d274" = 1.8
  dimension "d277" = 3.5
  dimension "d278" = 3.5
  dimension "d289" = 20
  dimension "d290" = 20
  measures "d273" diameter of A18
  measures "d274" diameter of A19
  measures "d277" distance of L0 A18.centre
  measures "d278" distance of L0 A19.centre
  measures "d289" horizontal distance of L3.end A19.centre
  measures "d290" horizontal distance of L1.start A18.centre
extrude "押し出し25" cut sketch "スケッチ20" against normal blind 6 contours A18 | A19 bodies 1
chamfer "面取り23" distance 0.5 angle 45 8 edges at (36, 112, 0) (-5.0839, 110.8219, 0) (-6.5, 52.75, 0) (-5.3219, -5.0839, 0) (36, -6.5, 0) (77.0839, -5.3219, 0) (78.5, 52.75, 0) (77.3219, 110.5839, 0) on bodies 1
sketch "スケッチ21" plane through (0, 0, 16) normal (0, 0, 1) x (-1, 0, 0)
  circle A0 centre (-7, -108.5) radius 0.9
  circle A1 centre (-65, -108.5) radius 0.9
  arc A2 (5.5, -86.5) -> (4.5, -85.5) centre (4.5, -86.5) ccw
  line L0 (4.5, -85.5) -> (-76.5, -85.5)
  arc A3 (-76.5, -85.5) -> (-77.5, -86.5) centre (-76.5, -86.5) ccw
  line L1 (-77.5, -86.5) -> (-77.5, -107)
  spline S0 degree 3 poles (-77.5, -107) (-77.5, -107.2964) (-77.4991, -107.5718) (-77.4694, -107.9483) (-77.4569, -108.0594) (-77.3918, -108.4745) (-77.3045, -108.8015) (-76.9308, -109.521) (-76.6724, -109.839) (-76.4029, -110.0896) (-76.1365, -110.3374) (-75.8631, -110.522) (-75.4373, -110.7274) (-75.2988, -110.7824) (-74.9267, -110.8989) (-74.7027, -110.9408) (-74.1654, -110.9986) (-73.8454, -111) (-73.5, -111) knots -0.679968 -0.679968 -0.679968 -0.679968 -0.591904 -0.591904 -0.55397 -0.55397 -0.448922 -0.448922 -0.339984 -0.339984 -0.339984 -0.2323 -0.2323 -0.182254 -0.182254 -0.103632 -0.103632 0 0 0 0
  line L2 (-73.5, -111) -> (1.5, -111)
  spline S1 degree 3 poles (1.5, -111) (1.7964, -111) (2.0718, -110.9991) (2.4483, -110.9694) (2.5594, -110.9569) (2.9745, -110.8918) (3.3015, -110.8045) (4.021, -110.4308) (4.339, -110.1724) (4.5896, -109.9029) (4.8374, -109.6365) (5.022, -109.3631) (5.2274, -108.9373) (5.2824, -108.7988) (5.3989, -108.4267) (5.4408, -108.2027) (5.4986, -107.6654) (5.5, -107.3454) (5.5, -107) knots -0.679968 -0.679968 -0.679968 -0.679968 -0.591904 -0.591904 -0.55397 -0.55397 -0.448922 -0.448922 -0.339984 -0.339984 -0.339984 -0.2323 -0.2323 -0.182254 -0.182254 -0.103632 -0.103632 0 0 0 0
  line L3 (5.5, -107) -> (5.5, -86.5)
  circle A4 centre (-7, -108.5) radius 1.1
  circle A5 centre (-65, -108.5) radius 1.1
  dimension "d285" = 2.2
  dimension "d286" = 2.2
  constraint concentric A0 A4
  constraint concentric A1 A5
  measures "d285" diameter of A4
  measures "d286" diameter of A5
extrude "押し出し26" cut sketch "スケッチ21" against normal blind 2 contours A4 | A5 bodies 2
sketch "スケッチ22" plane through (0, 0, 0) normal (0, 0, -1) x (1, 0, 0)
  circle A0 centre (36, -68) radius 2
  circle A1 centre (54, -51) radius 2
  circle A2 centre (18, -17) radius 2
  circle A3 centre (56.5, -4) radius 2
  circle A4 centre (18, -34) radius 2
  circle A5 centre (36, -51) radius 2
  circle A6 centre (54, -68) radius 2
  circle A7 centre (18, -68) radius 2
  circle A8 centre (54, -34) radius 2
  circle A9 centre (36, -17) radius 2
  circle A10 centre (54, -17) radius 2
  circle A11 centre (36, -34) radius 2
  circle A12 centre (18, -51) radius 2
  circle A13 centre (15.5, -4) radius 2
  circle A14 centre (-0.5, -106) radius 3.75
  circle A15 centre (-0.5, 0.5) radius 3.75
  circle A16 centre (72.5, -106) radius 3.75
  circle A17 centre (72.5, 0.5) radius 3.75
  circle A18 centre (13.5, -108.5) radius 0.9
  circle A19 centre (58.5, -108.5) radius 0.9
  spline S0 degree 3 poles (73.5, 6) (73.8454, 6) (74.1849, 5.9994) (74.7818, 5.9352) (75.0396, 5.8875) (75.4714, 5.7522) (75.6329, 5.6882) (76.1271, 5.4498) (76.4404, 5.2376) (76.7434, 4.9558) (77.05, 4.6706) (77.3444, 4.3096) (77.7773, 3.4759) (77.8795, 3.092) (77.9671, 2.5337) (77.9839, 2.3219) (77.9999, 1.9076) (78, 1.7055) (78, 1.5) knots 0 0 0 0 0.103632 0.103632 0.182254 0.182254 0.2323 0.2323 0.339984 0.339984 0.339984 0.448922 0.448922 0.55397 0.55397 0.618933 0.618933 0.679968 0.679968 0.679968 0.679968
  line L0 (73.5, 6) -> (-1.5, 6)
  spline S1 degree 3 poles (-6, 1.5) (-6, 1.8454) (-5.9994, 2.1849) (-5.9352, 2.7818) (-5.8875, 3.0396) (-5.7522, 3.4714) (-5.6882, 3.6329) (-5.4498, 4.1271) (-5.2376, 4.4404) (-4.9558, 4.7434) (-4.6706, 5.05) (-4.3096, 5.3444) (-3.4759, 5.7773) (-3.092, 5.8795) (-2.5337, 5.9671) (-2.3219, 5.9839) (-1.9076, 5.9999) (-1.7055, 6) (-1.5, 6) knots 0 0 0 0 0.103632 0.103632 0.182254 0.182254 0.2323 0.2323 0.339984 0.339984 0.339984 0.448922 0.448922 0.55397 0.55397 0.618933 0.618933 0.679968 0.679968 0.679968 0.679968
  line L1 (-6, 1.5) -> (-6, -107)
  spline S2 degree 3 poles (-1.5, -111.5) (-1.8454, -111.5) (-2.1849, -111.4994) (-2.7818, -111.4352) (-3.0396, -111.3875) (-3.4714, -111.2522) (-3.6329, -111.1882) (-4.1271, -110.9498) (-4.4404, -110.7376) (-4.7434, -110.4558) (-5.05, -110.1706) (-5.3444, -109.8096) (-5.7773, -108.9759) (-5.8795, -108.592) (-5.9671, -108.0337) (-5.9839, -107.8219) (-5.9999, -107.4076) (-6, -107.2055) (-6, -107) knots 0 0 0 0 0.103632 0.103632 0.182254 0.182254 0.2323 0.2323 0.339984 0.339984 0.339984 0.448922 0.448922 0.55397 0.55397 0.618933 0.618933 0.679968 0.679968 0.679968 0.679968
  line L2 (-2, -111.5) -> (74, -111.5)
  line L3 (74, -100.5) -> (-2, -100.5)
  line L4 (-6, -104.5) -> (-6, -107.5)
  line L5 (78, -104.5) -> (78, -107.5)
  line L6 (78, 1.5) -> (78, -107)
  arc A20 (-2, -100.5) -> (-6, -104.5) centre (-2, -104.5) ccw
  arc A21 (-6, -107.5) -> (-2, -111.5) centre (-2, -107.5) ccw
  arc A22 (78, -104.5) -> (74, -100.5) centre (74, -104.5) ccw
  arc A23 (74, -111.5) -> (78, -107.5) centre (74, -107.5) ccw
  point P0 (73.5, -111.5)
  point P1 (78, -107)
  dimension "d292" = 5.5
  dimension "d294" = 4
  dimension "d295" = 4
  dimension "d296" = 4
  dimension "d297" = 4
  constraint perpendicular L1 L3
  constraint perpendicular L3 L4
  constraint coincident L2 P0
  constraint coincident S2.start L2
  constraint coincident L5 P1
  constraint tangent L3 A20
  constraint tangent L4 A20
  constraint coincident L1.end L4
  constraint tangent L4 A21
  constraint tangent L2 A21
  constraint tangent L3 A22
  constraint tangent L5 A22
  constraint tangent L2 A23
  constraint tangent L5 A23
  measures "d292" distance of A14.centre L3
  measures "d294" radius of A20
  measures "d295" radius of A21
  measures "d296" radius of A22
  measures "d297" radius of A23
extrude "押し出し27" add sketch "スケッチ22" along normal blind 4 separate body contours A14 | A16 | L1 S2 L2 L3 L4 L5 L6 A20 A21 A22 A23 | S2 L4 A21 | S2 L2 A21 makes body 3
equation "d3 = ( 18 * 4 ) * 1 mm"
equation "d4 = ( 17 * 5 ) * 1 mm"
equation "d13 = 7 mm + 2 mm + 5 mm"
equation "d22 = -6.00 mm - 5 mm"
equation "d52 = ( 17 * 2 ) * 1 mm"
equation "d53 = ( 18 * 2 ) * 1 mm"
equation "d56 = ( 17 * 2 ) * 1 mm"
equation "d60 = ( 18 * 2 ) * 1 mm"
equation "d62 = ( 17 * 2 ) * 1 mm"
equation "d70 = ( 18 * 2 ) * 1 mm"
equation "d72 = ( 17 * 2 ) * 1 mm"
equation "d75 = ( 18 * 2 ) * 1 mm"
equation "d77 = ( 17 * 2 ) * 1 mm"
equation "d78 = ( 17 * 2 ) * 1 mm"
